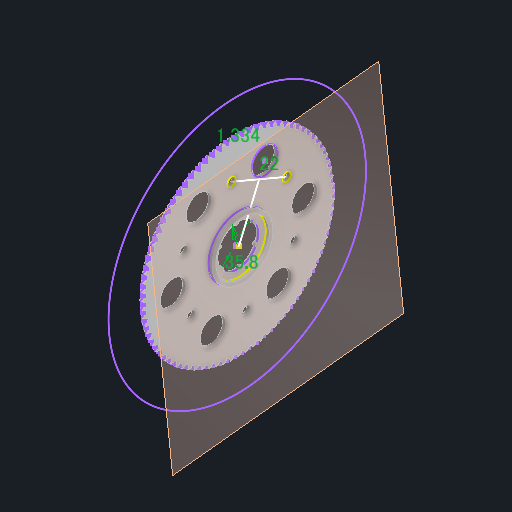
# Autodesk Inventor part: 25A80_()
Saved by Autodesk Inventor 2025.2 (Build 292293000, 293)
## iProperties
Category: PARTsolutions
Company: KANA
Created: 2025-03-15
Part Number: 25A80_()
Material: Generic
Catalog Web Link: www.cadenas.de
Description: 25A-Un-finished
Vendor: KANA
Document SubType Name: Modeling
Designer: psAdmin
Manufacturer: KANA
Mass: 58.7278 g
Surface Area: 427.105 cm^2
Volume: 58.7278 cm^3
Density: 1 g/cm^3
Appearance: PSOLRGB-175-175-175
PSOL_IDENT_0: {$CADENAS_DATA/23d-libs/kana/sprockets/chain_no_25/un_finished_sprocket_steel/a_type/25a.prj},156 {V
PSOL_IDENT_1: TYP=3D},{NB=25A80_()},{LINA=25A80},{NN=25A},{DATE=07.03.2025 00:51:20},{GEOMDATE=20.11.2024 07:31:23
PSOL_IDENT_2: },{VERSION=},{LINEID=550},{WBVAR=SURFT},{WBNUMERIC=}  {NB=25A80_()},{LINA=25A80},{KT=DUMMY},{ORDERNO=
PSOL_IDENT_3: 25A80},{TYPE=25A},{NOT=80},{NOTX=80.000},{DP=161.74},{DC=158.44},{DC2=158.44},{DO=165},{T=2.9},{DR=3
PSOL_IDENT_4: .300},{MAT=None},{MATC=},{SD=11},{SURFT=},{SURFTNB=},{DCX2=0},{CAUTION=The tooth profile in the CAD
PSOL_IDENT_5: models differ from the actual shape.}
NB: 25A80_()
NN: 25A
NT: Un-finished
NBSYN: 25A$NOT._($SURFT.)
LINA: 25A80
CATALOG: KANA
TYPE: 25A
NOT: 80
DP: 161.74
DC: 158.44
DC2: 158.44
DO: 165
T: 2.9
SD: 11
SURFT: No symbol : No
CAUTION: The tooth profile in the CAD models differ from the actual shape.
SUPPLIER: KANA
ARTICLENO: 25A80_()
BOMINFO: 25A80
CREATOR: CADENAS GmbH
Title: 25A80
Author: Cadenas PARTsolutions
Comments: Un-finished
Autodesk Inventor part; units mm, degrees
(part 1 of 2)
ref_plane "YZ Plane" through (0, 0, 0) normal (1, 0, 0) x (0, 1, 0)
ref_plane "XZ Plane" through (0, 0, 0) normal (0, 1, 0) x (-1, 0, 0)
ref_plane "XY Plane" through (0, 0, 0) normal (0, 0, 1) x (1, 0, 0)
sketch "Sketch_1" plane through (0, 0, 0) normal (0, 0, 1) x (1, 0, 0)
  line L0 (2.9, 0) -> (0, 0)
  line L1 (0, 5.5) -> (2.9, 5.5)
  line L2 (2.9, 5.5) -> (2.9, 81.2642)
  arc A0 (2.9, 81.2642) -> (2.175, 82.5) centre (-0.241, 80.2521) ccw
  line L3 (2.175, 82.5) -> (0.725, 82.5)
  arc A1 (0.725, 82.5) -> (0, 81.2642) centre (3.141, 80.2521) ccw
  line L4 (0, 81.2642) -> (0, 5.5)
  constraints: 10 end point, 4 point on circle, 2 centre point
revolve "Revolution1" add sketch "Sketch_1" angle 360 about axis through (2.9, 0, 0) along (1, 0, 0)
sketch "Sketch_2" plane through (1.45, 0, 0) normal (1, 0, 0) x (0, 0, -1)
  circle A0 centre (0, 0) radius 110
  arc A1 (-82.4999, 0.15) -> (-82.4999, -0.15) centre (0, 0) ccw
  line L0 (-82.4999, -0.15) -> (-79.9248, -1.781)
  arc A2 (-79.8181, -4.4953) -> (-79.9248, -1.781) centre (-80.8077, -3.1749) ccw
  line L1 (-79.8181, -4.4953) -> (-82.2573, -6.3233)
  arc A3 (-82.2573, -6.3233) -> (-82.2338, -6.6224) centre (0, 0) ccw
  line L2 (-82.2338, -6.6224) -> (-79.5387, -8.0464)
  arc A4 (-79.2194, -10.7439) -> (-79.5387, -8.0464) centre (-80.3094, -9.5053) ccw
  line L3 (-79.2194, -10.7439) -> (-81.5076, -12.7577)
  arc A5 (-81.5076, -12.7577) -> (-81.4607, -13.054) centre (0, 0) ccw
  line L4 (-81.4607, -13.054) -> (-78.6621, -14.2621)
  arc A6 (-78.1322, -16.9263) -> (-78.6621, -14.2621) centre (-79.3161, -15.777) ccw
  line L5 (-78.1322, -16.9263) -> (-80.2554, -19.1134)
  arc A7 (-80.2554, -19.1134) -> (-80.1854, -19.4051) centre (0, 0) ccw
  line L6 (-80.1854, -19.4051) -> (-77.3007, -20.3899)
  arc A8 (-76.5633, -23.0043) -> (-77.3007, -20.3899) centre (-77.8338, -21.9514) ccw
  line L7 (-76.5633, -23.0043) -> (-78.5084, -25.3512)
  arc A9 (-78.5084, -25.3512) -> (-78.4157, -25.6365) centre (0, 0) ccw
  line L8 (-78.4157, -25.6365) -> (-75.4626, -26.392)
  arc A10 (-74.5224, -28.9404) -> (-75.4626, -26.392) centre (-75.8715, -27.9905) ccw
  line L9 (-74.5224, -28.9404) -> (-76.2773, -31.4328)
  arc A11 (-76.2773, -31.4328) -> (-76.1625, -31.7099) centre (0, 0) ccw
  line L10 (-76.1625, -31.7099) -> (-73.1593, -32.2313)
  arc A12 (-72.0221, -34.6982) -> (-73.1593, -32.2313) centre (-73.4415, -33.857) ccw
  line L11 (-72.0221, -34.6982) -> (-73.576, -37.3205)
  arc A13 (-73.576, -37.3205) -> (-73.4398, -37.5878) centre (0, 0) ccw
  line L12 (-73.4398, -37.5878) -> (-70.4049, -37.872)
  arc A14 (-69.0776, -40.242) -> (-70.4049, -37.872) centre (-70.5588, -39.5148) ccw
  line L13 (-69.0776, -40.242) -> (-70.4211, -42.9782)
  arc A15 (-70.4211, -42.9782) -> (-70.2643, -43.234) centre (0, 0) ccw
  line L14 (-70.2643, -43.234) -> (-67.2165, -43.2791)
  arc A16 (-65.7074, -45.5377) -> (-67.2165, -43.2791) centre (-67.2409, -44.929) ccw
  line L15 (-65.7074, -45.5377) -> (-66.832, -48.3709)
  arc A17 (-66.832, -48.3709) -> (-66.6556, -48.6136) centre (0, 0) ccw
  line L16 (-66.6556, -48.6136) -> (-63.6136, -48.4195)
  arc A18 (-61.932, -50.5527) -> (-63.6136, -48.4195) centre (-63.5086, -50.0661) ccw
  line L17 (-61.932, -50.5527) -> (-62.8308, -53.4653)
  arc A19 (-62.8308, -53.4653) -> (-62.636, -53.6934) centre (0, 0) ccw
  line L18 (-62.636, -53.6934) -> (-59.6186, -53.2613)
  arc A20 (-57.7747, -55.256) -> (-59.6186, -53.2613) centre (-59.3847, -54.8946) ccw
  line L19 (-57.7747, -55.256) -> (-58.4423, -58.2302)
  arc A21 (-58.4423, -58.2302) -> (-58.2301, -58.4423) centre (0, 0) ccw
  line L20 (-58.2301, -58.4423) -> (-55.256, -57.7747)
  arc A22 (-53.2613, -59.6186) -> (-55.256, -57.7747) centre (-54.8946, -59.3847) ccw
  line L21 (-53.2613, -59.6186) -> (-53.6934, -62.636)
  arc A23 (-53.6934, -62.636) -> (-53.4653, -62.8308) centre (0, 0) ccw
  line L22 (-53.4653, -62.8308) -> (-50.5527, -61.932)
  arc A24 (-48.4195, -63.6136) -> (-50.5527, -61.932) centre (-50.0661, -63.5086) ccw
  line L23 (-48.4195, -63.6136) -> (-48.6136, -66.6556)
  arc A25 (-48.6136, -66.6556) -> (-48.3709, -66.832) centre (0, 0) ccw
  line L24 (-48.3709, -66.832) -> (-45.5377, -65.7074)
  arc A26 (-43.2791, -67.2165) -> (-45.5377, -65.7074) centre (-44.929, -67.241) ccw
  line L25 (-43.2791, -67.2165) -> (-43.234, -70.2643)
  arc A27 (-43.234, -70.2643) -> (-42.9782, -70.4211) centre (0, 0) ccw
  line L26 (-42.9782, -70.4211) -> (-40.242, -69.0777)
  arc A28 (-37.872, -70.4049) -> (-40.242, -69.0777) centre (-39.5148, -70.5588) ccw
  line L27 (-37.872, -70.4049) -> (-37.5878, -73.4398)
  arc A29 (-37.5878, -73.4398) -> (-37.3205, -73.576) centre (0, 0) ccw
  line L28 (-37.3205, -73.576) -> (-34.6982, -72.0221)
  arc A30 (-32.2313, -73.1593) -> (-34.6982, -72.0221) centre (-33.857, -73.4415) ccw
  line L29 (-32.2313, -73.1593) -> (-31.7099, -76.1625)
  arc A31 (-31.7099, -76.1625) -> (-31.4327, -76.2773) centre (0, 0) ccw
  line L30 (-31.4327, -76.2773) -> (-28.9404, -74.5224)
  arc A32 (-26.392, -75.4626) -> (-28.9404, -74.5224) centre (-27.9905, -75.8715) ccw
  line L31 (-26.392, -75.4626) -> (-25.6365, -78.4157)
  arc A33 (-25.6365, -78.4157) -> (-25.3512, -78.5084) centre (0, 0) ccw
  line L32 (-25.3512, -78.5084) -> (-23.0043, -76.5633)
  arc A34 (-20.3899, -77.3007) -> (-23.0043, -76.5633) centre (-21.9514, -77.8338) ccw
  line L33 (-20.3899, -77.3007) -> (-19.4051, -80.1854)
  arc A35 (-19.4051, -80.1854) -> (-19.1134, -80.2554) centre (0, 0) ccw
  line L34 (-19.1134, -80.2554) -> (-16.9263, -78.1322)
  arc A36 (-14.2621, -78.6622) -> (-16.9263, -78.1322) centre (-15.777, -79.3161) ccw
  line L35 (-14.2621, -78.6622) -> (-13.054, -81.4607)
  arc A37 (-13.054, -81.4607) -> (-12.7577, -81.5076) centre (0, 0) ccw
  line L36 (-12.7577, -81.5076) -> (-10.7439, -79.2194)
  arc A38 (-8.0464, -79.5387) -> (-10.7439, -79.2194) centre (-9.5052, -80.3095) ccw
  line L37 (-8.0464, -79.5387) -> (-6.6224, -82.2338)
  arc A39 (-6.6224, -82.2338) -> (-6.3233, -82.2573) centre (0, 0) ccw
  line L38 (-6.3233, -82.2573) -> (-4.4953, -79.8181)
  arc A40 (-1.781, -79.9248) -> (-4.4953, -79.8181) centre (-3.1749, -80.8077) ccw
  line L39 (-1.781, -79.9248) -> (-0.15, -82.4999)
  arc A41 (-0.15, -82.4999) -> (0.15, -82.4999) centre (0, 0) ccw
  line L40 (0.15, -82.4999) -> (1.781, -79.9248)
  arc A42 (4.4953, -79.8181) -> (1.781, -79.9248) centre (3.1749, -80.8077) ccw
  line L41 (4.4953, -79.8181) -> (6.3233, -82.2573)
  arc A43 (6.3233, -82.2573) -> (6.6224, -82.2338) centre (0, 0) ccw
  line L42 (6.6224, -82.2338) -> (8.0464, -79.5387)
  arc A44 (10.7439, -79.2194) -> (8.0464, -79.5387) centre (9.5052, -80.3095) ccw
  line L43 (10.7439, -79.2194) -> (12.7577, -81.5076)
  arc A45 (12.7577, -81.5076) -> (13.054, -81.4607) centre (0, 0) ccw
  line L44 (13.054, -81.4607) -> (14.2621, -78.6622)
  arc A46 (16.9263, -78.1322) -> (14.2621, -78.6622) centre (15.777, -79.3161) ccw
  line L45 (16.9263, -78.1322) -> (19.1134, -80.2554)
  arc A47 (19.1134, -80.2554) -> (19.4051, -80.1854) centre (0, 0) ccw
  line L46 (19.4051, -80.1854) -> (20.3899, -77.3007)
  arc A48 (23.0043, -76.5633) -> (20.3899, -77.3007) centre (21.9514, -77.8338) ccw
  line L47 (23.0043, -76.5633) -> (25.3512, -78.5084)
  arc A49 (25.3512, -78.5084) -> (25.6365, -78.4157) centre (0, 0) ccw
  line L48 (25.6365, -78.4157) -> (26.392, -75.4626)
  arc A50 (28.9404, -74.5224) -> (26.392, -75.4626) centre (27.9905, -75.8715) ccw
  line L49 (28.9404, -74.5224) -> (31.4327, -76.2773)
  arc A51 (31.4327, -76.2773) -> (31.7099, -76.1625) centre (0, 0) ccw
  line L50 (31.7099, -76.1625) -> (32.2313, -73.1593)
  arc A52 (34.6982, -72.0221) -> (32.2313, -73.1593) centre (33.857, -73.4415) ccw
  line L51 (34.6982, -72.0221) -> (37.3205, -73.576)
  arc A53 (37.3205, -73.576) -> (37.5878, -73.4398) centre (0, 0) ccw
  line L52 (37.5878, -73.4398) -> (37.872, -70.4049)
  arc A54 (40.242, -69.0777) -> (37.872, -70.4049) centre (39.5148, -70.5588) ccw
  line L53 (40.242, -69.0777) -> (42.9782, -70.4211)
  arc A55 (42.9782, -70.4211) -> (43.234, -70.2643) centre (0, 0) ccw
  line L54 (43.234, -70.2643) -> (43.2791, -67.2165)
  arc A56 (45.5377, -65.7074) -> (43.2791, -67.2165) centre (44.929, -67.241) ccw
  line L55 (45.5377, -65.7074) -> (48.3709, -66.832)
  arc A57 (48.3709, -66.832) -> (48.6136, -66.6556) centre (0, 0) ccw
  line L56 (48.6136, -66.6556) -> (48.4195, -63.6136)
  arc A58 (50.5527, -61.932) -> (48.4195, -63.6136) centre (50.0661, -63.5086) ccw
  line L57 (50.5527, -61.932) -> (53.4653, -62.8308)
  arc A59 (53.4653, -62.8308) -> (53.6934, -62.636) centre (0, 0) ccw
  line L58 (53.6934, -62.636) -> (53.2613, -59.6186)
  arc A60 (55.256, -57.7747) -> (53.2613, -59.6186) centre (54.8946, -59.3847) ccw
  line L59 (55.256, -57.7747) -> (58.2301, -58.4423)
  arc A61 (58.2301, -58.4423) -> (58.4423, -58.2302) centre (0, 0) ccw
  line L60 (58.4423, -58.2302) -> (57.7747, -55.256)
  arc A62 (59.6186, -53.2613) -> (57.7747, -55.256) centre (59.3847, -54.8946) ccw
  line L61 (59.6186, -53.2613) -> (62.636, -53.6934)
  arc A63 (62.636, -53.6934) -> (62.8308, -53.4653) centre (0, 0) ccw
  line L62 (62.8308, -53.4653) -> (61.932, -50.5527)
  arc A64 (63.6136, -48.4195) -> (61.932, -50.5527) centre (63.5086, -50.0661) ccw
  line L63 (63.6136, -48.4195) -> (66.6556, -48.6136)
  arc A65 (66.6556, -48.6136) -> (66.832, -48.3709) centre (0, 0) ccw
  line L64 (66.832, -48.3709) -> (65.7074, -45.5377)
  arc A66 (67.2165, -43.2791) -> (65.7074, -45.5377) centre (67.2409, -44.929) ccw
  line L65 (67.2165, -43.2791) -> (70.2643, -43.234)
  arc A67 (70.2643, -43.234) -> (70.4211, -42.9782) centre (0, 0) ccw
  line L66 (70.4211, -42.9782) -> (69.0776, -40.242)
  arc A68 (70.4049, -37.872) -> (69.0776, -40.242) centre (70.5588, -39.5148) ccw
  line L67 (70.4049, -37.872) -> (73.4398, -37.5878)
  arc A69 (73.4398, -37.5878) -> (73.576, -37.3205) centre (0, 0) ccw
  line L68 (73.576, -37.3205) -> (72.0221, -34.6982)
  arc A70 (73.1593, -32.2313) -> (72.0221, -34.6982) centre (73.4415, -33.857) ccw
  line L69 (73.1593, -32.2313) -> (76.1625, -31.7099)
  arc A71 (76.1625, -31.7099) -> (76.2773, -31.4328) centre (0, 0) ccw
  line L70 (76.2773, -31.4328) -> (74.5224, -28.9404)
  arc A72 (75.4626, -26.392) -> (74.5224, -28.9404) centre (75.8715, -27.9905) ccw
  line L71 (75.4626, -26.392) -> (78.4157, -25.6365)
  arc A73 (78.4157, -25.6365) -> (78.5084, -25.3512) centre (0, 0) ccw
  line L72 (78.5084, -25.3512) -> (76.5633, -23.0043)
  arc A74 (77.3007, -20.3899) -> (76.5633, -23.0043) centre (77.8338, -21.9514) ccw
  line L73 (77.3007, -20.3899) -> (80.1854, -19.4051)
  arc A75 (80.1854, -19.4051) -> (80.2554, -19.1134) centre (0, 0) ccw
  line L74 (80.2554, -19.1134) -> (78.1322, -16.9263)
  arc A76 (78.6621, -14.2621) -> (78.1322, -16.9263) centre (79.3161, -15.777) ccw
  line L75 (78.6621, -14.2621) -> (81.4607, -13.054)
  arc A77 (81.4607, -13.054) -> (81.5076, -12.7577) centre (0, 0) ccw
  line L76 (81.5076, -12.7577) -> (79.2194, -10.7439)
  arc A78 (79.5387, -8.0464) -> (79.2194, -10.7439) centre (80.3094, -9.5053) ccw
  line L77 (79.5387, -8.0464) -> (82.2338, -6.6224)
  arc A79 (82.2338, -6.6224) -> (82.2573, -6.3233) centre (0, 0) ccw
  line L78 (82.2573, -6.3233) -> (79.8181, -4.4953)
  arc A80 (79.9248, -1.781) -> (79.8181, -4.4953) centre (80.8077, -3.1749) ccw
  line L79 (79.9248, -1.781) -> (82.4999, -0.15)
  arc A81 (82.4999, -0.15) -> (82.4999, 0.15) centre (0, 0) ccw
  line L80 (82.4999, 0.15) -> (79.9248, 1.781)
  arc A82 (79.0225, 3.671) -> (79.9248, 1.781) centre (80.6244, 3.2753) ccw
  line L81 (79.0225, 3.671) -> (81.4805, 5.4737)
  arc A83 (81.4805, 5.4737) -> (81.46, 5.773) centre (-0.8378, 0.0009) ccw
  line L82 (81.46, 5.773) -> (78.7798, 7.2248)
  arc A84 (78.4884, 9.9255) -> (78.7798, 7.2248) centre (79.5656, 8.6756) ccw
  line L83 (78.4884, 9.9255) -> (80.7973, 11.9155)
  arc A85 (80.7973, 11.9155) -> (80.7535, 12.2122) centre (-0.8378, 0.0009) ccw
  line L84 (80.7535, 12.2122) -> (77.9676, 13.4492)
  arc A86 (77.4652, 16.1187) -> (77.9676, 13.4492) centre (78.6371, 14.9572) ccw
  line L85 (77.4652, 16.1187) -> (79.6109, 18.2838)
  arc A87 (79.6109, 18.2838) -> (79.5439, 18.5762) centre (-0.8378, 0.0009) ccw
  line L86 (79.5439, 18.5762) -> (76.6695, 19.5908)
  arc A88 (75.9592, 22.2126) -> (76.6695, 19.5908) centre (77.2187, 21.1467) ccw
  line L87 (75.9592, 22.2126) -> (77.9284, 24.5393)
  arc A89 (77.9284, 24.5393) -> (77.8387, 24.8256) centre (-0.8378, 0.0009) ccw
  line L88 (77.8387, 24.8256) -> (74.8936, 25.6115)
  arc A90 (73.9798, 28.1696) -> (74.8936, 25.6115) centre (75.319, 27.2057) ccw
  line L89 (73.9798, 28.1696) -> (75.7604, 30.6436)
  arc A91 (75.7604, 30.6436) -> (75.6484, 30.9219) centre (-0.8378, 0.0009) ccw
  line L90 (75.6484, 30.9219) -> (72.6507, 31.4744)
  arc A92 (71.539, 33.9529) -> (72.6507, 31.4744) centre (72.9498, 33.0971) ccw
  line L91 (71.539, 33.9529) -> (73.12, 36.559)
  arc A93 (73.12, 36.559) -> (72.9866, 36.8277) centre (-0.8378, 0.0009) ccw
  line L92 (72.9866, 36.8277) -> (69.9548, 37.1432)
  arc A94 (68.6521, 39.5268) -> (69.9548, 37.1432) centre (70.1256, 38.7843) ccw
  line L93 (68.6521, 39.5268) -> (70.0237, 42.2489)
  arc A95 (70.0237, 42.2489) -> (69.8696, 42.5063) centre (-0.8378, 0.0009) ccw
  line L94 (69.8696, 42.5063) -> (66.8224, 42.583)
  arc A96 (65.3367, 44.8571) -> (66.8224, 42.583) centre (66.8639, 44.2325) ccw
  line L95 (65.3367, 44.8571) -> (66.4905, 47.6784)
  arc A97 (66.4905, 47.6784) -> (66.3167, 47.9229) centre (-0.8378, 0.0009) ccw
  line L96 (66.3167, 47.9229) -> (63.2729, 47.7603)
  arc A98 (61.6133, 49.9108) -> (63.2729, 47.7603) centre (63.1849, 49.408) ccw
  line L97 (61.6133, 49.9108) -> (62.5425, 52.8149)
  arc A99 (62.5425, 52.8149) -> (62.3498, 53.0441) centre (-0.5024, 0) ccw
  line L98 (62.3498, 53.0441) -> (59.3281, 52.6432)
  arc A100 (57.5049, 54.6568) -> (59.3281, 52.6432) centre (59.1111, 54.2788) ccw
  line L99 (57.5049, 54.6568) -> (58.2032, 57.6239)
  arc A101 (58.2032, 57.6239) -> (57.9933, 57.8382) centre (-0.8378, 0.0009) ccw
  line L100 (57.9933, 57.8382) -> (55.0124, 57.2014)
  arc A102 (53.0368, 59.0658) -> (55.0124, 57.2014) centre (54.6677, 58.815) ccw
  line L101 (53.0368, 59.0658) -> (53.5002, 62.0786)
  arc A103 (53.5002, 62.0786) -> (53.2741, 62.2758) centre (-0.8378, 0.0009) ccw
  line L102 (53.2741, 62.2758) -> (50.3523, 61.4071)
  arc A104 (48.2366, 63.1107) -> (50.3523, 61.4071) centre (49.8821, 62.9886) ccw
  line L103 (48.2366, 63.1107) -> (48.4621, 66.1505)
  arc A105 (48.4621, 66.1505) -> (48.2212, 66.3294) centre (-0.8378, 0.0009) ccw
  line L104 (48.2212, 66.3294) -> (45.3766, 65.2341)
  arc A106 (43.1338, 66.7665) -> (45.3766, 65.2341) centre (44.7837, 66.7739) ccw
  line L105 (43.1338, 66.7665) -> (43.1201, 69.8146)
  arc A107 (43.1201, 69.8146) -> (42.8659, 69.974) centre (-0.8378, 0.0009) ccw
  line L106 (42.8659, 69.974) -> (40.116, 68.6589)
  arc A108 (37.7598, 70.0106) -> (40.116, 68.6589) centre (39.4042, 70.1475) ccw
  line L107 (37.7598, 70.0106) -> (37.507, 73.0483)
  arc A109 (37.507, 73.0483) -> (37.2412, 73.1873) centre (-0.8378, 0.0009) ccw
  line L108 (37.2412, 73.1873) -> (34.6029, 71.6605)
  arc A110 (32.148, 72.8232) -> (34.6029, 71.6605) centre (33.7765, 73.0886) ccw
  line L109 (32.148, 72.8232) -> (31.6576, 75.8316)
  arc A111 (31.6576, 75.8316) -> (31.3816, 75.9493) centre (-0.8378, 0.0009) ccw
  line L110 (31.3816, 75.9493) -> (28.8713, 74.2202)
  arc A112 (26.3327, 75.1867) -> (28.8713, 74.2202) centre (27.9354, 75.5791) ccw
  line L111 (26.3327, 75.1867) -> (25.6078, 78.1474)
  arc A113 (25.6078, 78.1474) -> (25.3235, 78.2431) centre (-0.8378, 0.0009) ccw
  line L112 (25.3235, 78.2431) -> (22.9566, 76.3224)
  arc A114 (20.3499, 77.0867) -> (22.9566, 76.3224) centre (21.9169, 77.6036) ccw
  line L113 (20.3499, 77.0867) -> (19.395, 79.9814)
  arc A115 (19.395, 79.9814) -> (19.104, 80.0545) centre (-0.8378, 0.0009) ccw
  line L114 (19.104, 80.0545) -> (16.8951, 77.954)
  arc A116 (14.2365, 78.5114) -> (16.8951, 77.954) centre (15.7581, 79.1497) ccw
  line L115 (14.2365, 78.5114) -> (13.0574, 81.3223)
  arc A117 (13.0574, 81.3223) -> (12.7616, 81.3723) centre (-0.8378, 0.0009) ccw
  line L116 (12.7616, 81.3723) -> (10.7243, 79.105)
  arc A118 (8.0302, 79.4521) -> (10.7243, 79.105) centre (9.497, 80.2078) ccw
  line L117 (8.0302, 79.4521) -> (6.6342, 82.1618)
  arc A119 (6.6342, 82.1618) -> (6.3354, 82.1885) centre (-0.8378, 0.0009) ccw
  line L118 (6.3354, 82.1885) -> (4.4822, 79.7683)
  arc A120 (1.7692, 79.903) -> (4.4822, 79.7683) centre (3.1722, 80.7714) ccw
  line L119 (1.7692, 79.903) -> (0.1649, 82.4948)
  arc A121 (0.1649, 82.4948) -> (-0.15, 82.4999) centre (-1.3174, 0.0081) ccw
  line L120 (-0.15, 82.4999) -> (-1.781, 79.9248)
  arc A122 (-4.4953, 79.8181) -> (-1.781, 79.9248) centre (-3.1749, 80.8077) ccw
  line L121 (-4.4953, 79.8181) -> (-6.3233, 82.2573)
  arc A123 (-6.3233, 82.2573) -> (-6.6224, 82.2338) centre (0, 0) ccw
  line L122 (-6.6224, 82.2338) -> (-8.0464, 79.5386)
  arc A124 (-10.7439, 79.2194) -> (-8.0464, 79.5386) centre (-9.5052, 80.3094) ccw
  line L123 (-10.7439, 79.2194) -> (-12.7577, 81.5076)
  arc A125 (-12.7577, 81.5076) -> (-13.054, 81.4607) centre (0, 0) ccw
  line L124 (-13.054, 81.4607) -> (-14.2621, 78.6621)
  arc A126 (-16.9263, 78.1322) -> (-14.2621, 78.6621) centre (-15.777, 79.3161) ccw
  line L125 (-16.9263, 78.1322) -> (-19.1134, 80.2554)
  arc A127 (-19.1134, 80.2554) -> (-19.4051, 80.1854) centre (0, 0) ccw
  line L126 (-19.4051, 80.1854) -> (-20.3899, 77.3007)
  arc A128 (-23.0043, 76.5633) -> (-20.3899, 77.3007) centre (-21.9514, 77.8338) ccw
  line L127 (-23.0043, 76.5633) -> (-25.3512, 78.5084)
  arc A129 (-25.3512, 78.5084) -> (-25.6365, 78.4157) centre (0, 0) ccw
  line L128 (-25.6365, 78.4157) -> (-26.392, 75.4626)
  arc A130 (-28.9404, 74.5224) -> (-26.392, 75.4626) centre (-27.9905, 75.8715) ccw
  line L129 (-28.9404, 74.5224) -> (-31.4327, 76.2773)
  arc A131 (-31.4327, 76.2773) -> (-31.7099, 76.1625) centre (0, 0) ccw
  line L130 (-31.7099, 76.1625) -> (-32.2313, 73.1593)
  arc A132 (-34.6982, 72.0221) -> (-32.2313, 73.1593) centre (-33.857, 73.4415) ccw
  line L131 (-34.6982, 72.0221) -> (-37.3205, 73.576)
  arc A133 (-37.3205, 73.576) -> (-37.5878, 73.4398) centre (0, 0) ccw
  line L132 (-37.5878, 73.4398) -> (-37.872, 70.4049)
  arc A134 (-40.242, 69.0776) -> (-37.872, 70.4049) centre (-39.5148, 70.5588) ccw
  line L133 (-40.242, 69.0776) -> (-42.9782, 70.4211)
  arc A135 (-42.9782, 70.4211) -> (-43.234, 70.2643) centre (0, 0) ccw
  line L134 (-43.234, 70.2643) -> (-43.2791, 67.2165)
  arc A136 (-45.5377, 65.7074) -> (-43.2791, 67.2165) centre (-44.929, 67.2409) ccw
  line L135 (-45.5377, 65.7074) -> (-48.3709, 66.832)
  arc A137 (-48.3709, 66.832) -> (-48.6136, 66.6556) centre (0, 0) ccw
  line L136 (-48.6136, 66.6556) -> (-48.4195, 63.6136)
  arc A138 (-50.5527, 61.9319) -> (-48.4195, 63.6136) centre (-50.0661, 63.5086) ccw
  line L137 (-50.5527, 61.9319) -> (-53.4653, 62.8308)
  arc A139 (-53.4653, 62.8308) -> (-53.6934, 62.636) centre (0, 0) ccw
  line L138 (-53.6934, 62.636) -> (-53.2613, 59.6186)
  arc A140 (-55.256, 57.7747) -> (-53.2613, 59.6186) centre (-54.8946, 59.3847) ccw
  line L139 (-55.256, 57.7747) -> (-58.2301, 58.4423)
  arc A141 (-58.2301, 58.4423) -> (-58.4423, 58.2301) centre (0, 0) ccw
  line L140 (-58.4423, 58.2301) -> (-57.7747, 55.256)
  arc A142 (-59.6186, 53.2613) -> (-57.7747, 55.256) centre (-59.3847, 54.8946) ccw
  line L141 (-59.6186, 53.2613) -> (-62.636, 53.6934)
  arc A143 (-62.636, 53.6934) -> (-62.8308, 53.4653) centre (0, 0) ccw
  line L142 (-62.8308, 53.4653) -> (-61.932, 50.5527)
  arc A144 (-63.6136, 48.4195) -> (-61.932, 50.5527) centre (-63.5086, 50.0661) ccw
  line L143 (-63.6136, 48.4195) -> (-66.6556, 48.6136)
  arc A145 (-66.6556, 48.6136) -> (-66.832, 48.3708) centre (0, 0) ccw
  line L144 (-66.832, 48.3708) -> (-65.7074, 45.5377)
  arc A146 (-67.2165, 43.2791) -> (-65.7074, 45.5377) centre (-67.2409, 44.929) ccw
  line L145 (-67.2165, 43.2791) -> (-70.2643, 43.234)
  arc A147 (-70.2643, 43.234) -> (-70.4211, 42.9782) centre (0, 0) ccw
  line L146 (-70.4211, 42.9782) -> (-69.0776, 40.242)
  arc A148 (-70.4049, 37.872) -> (-69.0776, 40.242) centre (-70.5588, 39.5148) ccw
  line L147 (-70.4049, 37.872) -> (-73.4398, 37.5878)
  arc A149 (-73.4398, 37.5878) -> (-73.576, 37.3205) centre (0, 0) ccw
  line L148 (-73.576, 37.3205) -> (-72.0221, 34.6982)
  arc A150 (-73.1593, 32.2313) -> (-72.0221, 34.6982) centre (-73.4415, 33.857) ccw
  line L149 (-73.1593, 32.2313) -> (-76.1625, 31.7099)
  arc A151 (-76.1625, 31.7099) -> (-76.2773, 31.4327) centre (0, 0) ccw
  line L150 (-76.2773, 31.4327) -> (-74.5224, 28.9404)
  arc A152 (-75.4626, 26.392) -> (-74.5224, 28.9404) centre (-75.8715, 27.9905) ccw
  line L151 (-75.4626, 26.392) -> (-78.4157, 25.6365)
  arc A153 (-78.4157, 25.6365) -> (-78.5084, 25.3512) centre (0, 0) ccw
  line L152 (-78.5084, 25.3512) -> (-76.5633, 23.0043)
  arc A154 (-77.3007, 20.3899) -> (-76.5633, 23.0043) centre (-77.8338, 21.9514) ccw
  line L153 (-77.3007, 20.3899) -> (-80.1854, 19.4051)
  arc A155 (-80.1854, 19.4051) -> (-80.2554, 19.1134) centre (0, 0) ccw
  line L154 (-80.2554, 19.1134) -> (-78.1322, 16.9263)
  arc A156 (-78.6621, 14.2621) -> (-78.1322, 16.9263) centre (-79.3161, 15.777) ccw
  line L155 (-78.6621, 14.2621) -> (-81.4607, 13.054)
  arc A157 (-81.4607, 13.054) -> (-81.5076, 12.7577) centre (0, 0) ccw
  line L156 (-81.5076, 12.7577) -> (-79.2194, 10.7439)
  arc A158 (-79.5387, 8.0464) -> (-79.2194, 10.7439) centre (-80.3094, 9.5052) ccw
  line L157 (-79.5387, 8.0464) -> (-82.2338, 6.6224)
  arc A159 (-82.2338, 6.6224) -> (-82.2573, 6.3233) centre (0, 0) ccw
  line L158 (-82.2573, 6.3233) -> (-79.8181, 4.4953)
  arc A160 (-79.9248, 1.781) -> (-79.8181, 4.4953) centre (-80.8077, 3.1749) ccw
  line L159 (-79.9248, 1.781) -> (-82.4999, 0.15)
  arc A161 (0.667, 81.6835) -> (-0.667, 81.6835) centre (0, 0) ccw
  circle A162 centre (0, 0) radius 17.9
  line L160 (-0.3663, 82.1584) -> (0.3731, 82.1584)
  dimension "d5" = 1.3341
  dimension "d19" = 35.8
  constraints: 322 end point, 322 point on circle, 163 centre point, 4 point on line, 2 coincident, 1 horizontal
  measures "d5" distance of A161.start A161.end
  measures "d19" diameter of A162
extrude "Extrusion1" cut sketch "Sketch_2" along normal mid plane 3.3 contours A0
ref_plane "Body_XY" through (0, 0, 0) normal (1, 0, 0) x (0, 0, -1)
ref_plane "Body_YZ" through (0, 0, 0) normal (0, 0, -1) x (0, 1, 0)
ref_plane "Body_ZX" through (0, 0, 0) normal (0, 1, 0) x (1, 0, 0)
sketch "スケッチ3" plane through (2.9, 8.6756, -79.5656) normal (1, 0, 0) x (0, 0.1072674, -0.9942302)
  circle A0 centre (-80.0371, -0.0908) radius 5.5 projected
  line L0 (-1.0768, -4.9175) -> (1.1501, -3.6267) projected
  arc A1 (1.1501, -3.6267) -> (1.1812, -2.8194) centre (-80.0371, -0.0908) ccw projected
  line L1 (1.1812, -2.8194) -> (-0.9369, -1.3582) projected
  arc A2 (-0.9369, 1.3582) -> (-0.9369, -1.3582) centre (0, 0) ccw projected
  line L2 (-0.9369, 1.3582) -> (1.1751, 2.8151) projected
  arc A3 (1.1751, 2.8151) -> (1.1417, 3.6315) centre (-80.0371, -0.0908) ccw projected
  line L3 (1.1417, 3.6315) -> (-1.0768, 4.9175) projected
  arc A4 (-1.2899, 7.6255) -> (-1.0768, 4.9175) centre (-0.2493, 6.345) ccw projected
  line L4 (-1.2899, 7.6255) -> (0.6902, 9.2346) projected
  arc A5 (0.6902, 9.2346) -> (0.5904, 10.0614) centre (-80.0371, -0.0908) ccw projected
  line L5 (0.5904, 10.0614) -> (-1.7086, 11.1628) projected
  arc A6 (-2.1335, 13.8457) -> (-1.7086, 11.1628) centre (-0.9956, 12.6509) ccw projected
  line L6 (-2.1335, 13.8457) -> (-0.3005, 15.5913) projected
  arc A7 (-0.3005, 15.5913) -> (-0.4698, 16.4293) centre (-80.0371, -0.0908) ccw projected
  line L7 (-0.4698, 16.4293) -> (-2.8284, 17.3393) projected
  arc A8 (-3.4625, 19.9807) -> (-2.8284, 17.3393) centre (-2.2344, 18.8787) ccw projected
  line L8 (-3.4625, 19.9807) -> (-1.7896, 21.8452) projected
  arc A9 (-1.7896, 21.8452) -> (-2.0327, 22.6945) centre (-80.0371, -0.0908) ccw projected
  line L9 (-2.0327, 22.6945) -> (-4.4294, 23.409) projected
  arc A10 (-5.2688, 25.9924) -> (-4.4294, 23.409) centre (-3.9581, 24.9902) ccw projected
  line L10 (-5.2688, 25.9924) -> (-3.7667, 27.9571) projected
  arc A11 (-3.7667, 27.9571) -> (-4.0884, 28.8169) centre (-80.0371, -0.0908) ccw projected
  line L11 (-4.0884, 28.8169) -> (-6.5017, 29.3343) projected
  arc A12 (-7.5412, 31.8439) -> (-6.5017, 29.3343) centre (-6.1559, 30.9476) ccw projected
  line L12 (-7.5412, 31.8439) -> (-6.2182, 33.889) projected
  arc A13 (-6.2182, 33.889) -> (-6.6241, 34.7574) centre (-80.0371, -0.0908) ccw projected
  line L13 (-6.6241, 34.7574) -> (-9.0325, 35.0787) projected
  arc A14 (-10.2657, 37.499) -> (-9.0325, 35.0787) centre (-8.8143, 36.7142) ccw projected
  line L14 (-10.2657, 37.499) -> (-9.1275, 39.6041) projected
  arc A15 (-9.1275, 39.6041) -> (-9.6237, 40.4779) centre (-80.0371, -0.0908) ccw projected
  line L15 (-9.6237, 40.4779) -> (-12.0062, 40.6069) projected
  arc A16 (-13.4255, 42.923) -> (-12.0062, 40.6069) centre (-11.917, 42.2545) ccw projected
  line L16 (-13.4255, 42.923) -> (-12.4752, 45.0673) projected
  arc A17 (-12.4752, 45.0673) -> (-13.068, 45.9418) centre (-80.0371, -0.0908) ccw projected
  line L17 (-13.068, 45.9418) -> (-15.4045, 45.8847) projected
  arc A18 (-17.0011, 48.0823) -> (-15.4045, 45.8847) centre (-15.4448, 47.5342) ccw projected
  line L18 (-17.0011, 48.0823) -> (-16.2394, 50.2452) projected
  arc A19 (-16.2394, 50.2452) -> (-16.9348, 51.1144) centre (-80.0371, -0.0908) ccw projected
  line L19 (-16.9348, 51.1144) -> (-19.2063, 50.8796) projected
  arc A20 (-20.9705, 52.9451) -> (-19.2063, 50.8796) centre (-19.376, 52.5209) ccw projected
  line L20 (-20.9705, 52.9451) -> (-20.3954, 55.1064) projected
  arc A21 (-20.3954, 55.1064) -> (-21.1994, 55.9626) centre (-80.0371, -0.0908) ccw projected
  line L21 (-21.1994, 55.9626) -> (-23.3884, 55.5608) projected
  arc A22 (-25.3092, 57.4816) -> (-23.3884, 55.5608) centre (-23.6863, 57.1837) ccw projected
  line L22 (-25.3092, 57.4816) -> (-24.9164, 59.6216) projected
  arc A23 (-24.9164, 59.6216) -> (-25.8341, 60.4559) centre (-80.0371, -0.0908) ccw projected
  line L23 (-25.8341, 60.4559) -> (-27.9249, 59.8995) projected
  arc A24 (-29.9904, 61.6637) -> (-27.9249, 59.8995) centre (-28.3491, 61.494) ccw projected
  line L24 (-29.9904, 61.6637) -> (-29.7733, 63.7639) projected
  arc A25 (-29.7733, 63.7639) -> (-30.809, 64.5657) centre (-80.0371, -0.0908) ccw projected
  line L25 (-30.809, 64.5657) -> (-32.7877, 63.8689) projected
  arc A26 (-34.9853, 65.4655) -> (-32.7877, 63.8689) centre (-33.3358, 65.4252) ccw projected
  line L26 (-34.9853, 65.4655) -> (-34.9354, 67.5088) projected
  arc A27 (-34.9354, 67.5088) -> (-36.0922, 68.2665) centre (-80.0371, -0.0908) ccw projected
  line L27 (-36.0922, 68.2665) -> (-37.947, 67.4445) projected
  arc A28 (-40.2631, 68.8638) -> (-37.947, 67.4445) centre (-38.6155, 68.953) ccw projected
  line L28 (-40.2631, 68.8638) -> (-40.3698, 70.8343) projected
  arc A29 (-40.3698, 70.8343) -> (-41.6496, 71.5351) centre (-80.0371, -0.0908) ccw projected
  line L29 (-41.6496, 71.5351) -> (-43.371, 70.6043) projected
  arc A30 (-45.7913, 71.8375) -> (-43.371, 70.6043) centre (-44.1558, 72.0557) ccw projected
  line L30 (-45.7913, 71.8375) -> (-46.0427, 73.7214) projected
  arc A31 (-46.0427, 73.7214) -> (-47.4454, 74.3514) centre (-80.0371, -0.0908) ccw projected
  line L31 (-47.4454, 74.3514) -> (-49.0261, 73.3288) projected
  arc A32 (-51.5357, 74.3683) -> (-49.0261, 73.3288) centre (-49.9224, 74.7141) ccw projected
  line L32 (-51.5357, 74.3683) -> (-51.9185, 76.1536) projected
  arc A33 (-51.9185, 76.1536) -> (-53.4424, 76.6985) centre (-80.0371, -0.0908) ccw projected
  line L33 (-53.4424, 76.6985) -> (-54.8776, 75.6012) projected
  arc A34 (-57.461, 76.4406) -> (-54.8776, 75.6012) centre (-55.8798, 76.9119) ccw projected
  line L34 (-57.461, 76.4406) -> (-57.9609, 78.1173) projected
  arc A35 (-57.9609, 78.1173) -> (-59.6024, 78.5622) centre (-80.0371, -0.0908) ccw projected
  line L35 (-59.6024, 78.5622) -> (-60.8893, 77.4075) projected
  arc A36 (-63.5307, 78.0416) -> (-60.8893, 77.4075) centre (-61.9913, 78.6356) ccw projected
  line L36 (-63.5307, 78.0416) -> (-64.1327, 79.6019) projected
  arc A37 (-64.1327, 79.6019) -> (-65.886, 79.9318) centre (-80.0371, -0.0908) ccw projected
  line L37 (-65.886, 79.9318) -> (-67.0243, 78.7365) projected
  arc A38 (-69.7072, 79.1614) -> (-67.0243, 78.7365) centre (-68.2191, 79.8744) ccw projected
  line L38 (-69.7072, 79.1614) -> (-70.3962, 80.5995) projected
  arc A39 (-70.3962, 80.5995) -> (-72.2514, 80.7996) centre (-80.0371, -0.0908) ccw projected
  line L39 (-72.2514, 80.7996) -> (-73.2346, 79.5639) projected
  arc A40 (-75.9446, 79.749) -> (-73.2346, 79.5639) centre (-74.5257, 80.5912) ccw projected
  line L40 (-75.9446, 79.749) -> (-76.7506, 81.1069) projected
  arc A41 (-76.7506, 81.1069) -> (-78.622, 81.1611) centre (-80.0371, -0.0908) ccw projected
  line L41 (-78.622, 81.1611) -> (-79.5052, 79.8521) projected
  arc A42 (-82.2214, 79.824) -> (-79.5052, 79.8521) centre (-80.873, 80.7749) ccw projected
  line L42 (-82.2214, 79.824) -> (-83.1315, 81.1145) projected
  arc A43 (-83.1315, 81.1145) -> (-85.0013, 81.0217) centre (-80.0371, -0.0908) ccw projected
  line L43 (-85.0013, 81.0217) -> (-85.7791, 79.6474) projected
  arc A44 (-88.4847, 79.4063) -> (-85.7791, 79.6474) centre (-87.215, 80.4601) ccw projected
  line L44 (-88.4847, 79.4063) -> (-89.4932, 80.6214) projected
  arc A45 (-89.4932, 80.6214) -> (-91.35, 80.3821) centre (-80.0371, -0.0908) ccw projected
  line L45 (-91.35, 80.3821) -> (-92.0175, 78.9511) projected
  arc A46 (-94.6959, 78.4984) -> (-92.0175, 78.9511) centre (-93.5129, 79.6486) ccw projected
  line L46 (-94.6959, 78.4984) -> (-95.7967, 79.6307) projected
  arc A47 (-95.7967, 79.6307) -> (-97.629, 79.2465) centre (-80.0371, -0.0908) ccw projected
  line L47 (-97.629, 79.2465) -> (-98.1822, 77.7674) projected
  arc A48 (-100.8168, 77.106) -> (-98.1822, 77.7674) centre (-99.7276, 78.3455) ccw projected
  line L48 (-100.8168, 77.106) -> (-102.0029, 78.1484) projected
  arc A49 (-102.0029, 78.1484) -> (-103.7995, 77.6217) centre (-80.0371, -0.0908) ccw projected
  line L49 (-103.7995, 77.6217) -> (-104.2349, 76.1038) projected
  arc A50 (-106.8095, 75.2377) -> (-104.2349, 76.1038) centre (-105.8209, 76.5588) ccw projected
  line L50 (-106.8095, 75.2377) -> (-108.0738, 76.1838) projected
  arc A51 (-108.0738, 76.1838) -> (-109.8235, 75.5177) centre (-80.0371, -0.0908) ccw projected
  line L51 (-109.8235, 75.5177) -> (-110.1385, 73.9704) projected
  arc A52 (-112.6372, 72.905) -> (-110.1385, 73.9704) centre (-111.7553, 74.2995) ccw projected
  line L52 (-112.6372, 72.905) -> (-113.9718, 73.749) projected
  arc A53 (-113.9718, 73.749) -> (-115.6638, 72.9476) centre (-80.0371, -0.0908) ccw projected
  line L53 (-115.6638, 72.9476) -> (-115.8564, 71.3803) projected
  arc A54 (-118.2639, 70.1222) -> (-115.8564, 71.3803) centre (-117.4941, 71.5816) ccw projected
  line L54 (-118.2639, 70.1222) -> (-119.6606, 70.8589) projected
  arc A55 (-119.6606, 70.8589) -> (-121.2845, 69.9273) centre (-80.0371, -0.0908) ccw projected
  line L55 (-121.2845, 69.9273) -> (-121.3536, 68.3497) projected
  arc A56 (-123.6549, 66.9065) -> (-121.3536, 68.3497) centre (-123.002, 68.4219) ccw projected
  line L56 (-123.6549, 66.9065) -> (-125.1051, 67.5313) projected
  arc A57 (-125.1051, 67.5313) -> (-126.6509, 66.4752) centre (-80.0371, -0.0908) ccw projected
  line L57 (-126.6509, 66.4752) -> (-126.596, 64.897) projected
  arc A58 (-128.777, 63.2778) -> (-126.596, 64.897) centre (-128.245, 64.8397) ccw projected
  line L58 (-128.777, 63.2778) -> (-130.2717, 63.7869) projected
  arc A59 (-130.2717, 63.7869) -> (-131.7299, 62.6127) centre (-80.0371, -0.0908) ccw projected
  line L59 (-131.7299, 62.6127) -> (-131.5514, 61.0437) projected
  arc A60 (-133.5986, 59.2583) -> (-131.5514, 61.0437) centre (-133.1908, 60.8572) ccw projected
  line L60 (-133.5986, 59.2583) -> (-135.1287, 59.6486) projected
  arc A61 (-135.1287, 59.6486) -> (-136.4902, 58.3636) centre (-80.0371, -0.0908) ccw projected
  line L61 (-136.4902, 58.3636) -> (-136.1891, 56.8135) projected
  arc A62 (-138.0899, 54.873) -> (-136.1891, 56.8135) centre (-137.8088, 56.4989) ccw projected
  line L62 (-138.0899, 54.873) -> (-139.6459, 55.142) projected
  arc A63 (-139.6459, 55.142) -> (-140.9025, 53.7542) centre (-80.0371, -0.0908) ccw projected
  line L63 (-140.9025, 53.7542) -> (-140.4807, 52.2325) projected
  arc A64 (-142.2234, 50.1488) -> (-140.4807, 52.2325) centre (-142.0707, 51.7917) ccw projected
  line L64 (-142.2234, 50.1488) -> (-143.7957, 50.2949) projected
  arc A65 (-143.7957, 50.2949) -> (-144.9395, 48.8128) centre (-80.0371, -0.0908) ccw projected
  line L65 (-144.9395, 48.8128) -> (-144.3996, 47.3288) projected
  arc A66 (-145.9734, 45.1149) -> (-144.3996, 47.3288) centre (-145.9501, 46.7647) ccw projected
  line L66 (-145.9734, 45.1149) -> (-147.5524, 45.1371) projected
  arc A67 (-147.5524, 45.1371) -> (-148.5763, 43.5698) centre (-80.0371, -0.0908) ccw projected
  line L67 (-148.5763, 43.5698) -> (-147.9217, 42.1328) projected
  arc A68 (-149.317, 39.8022) -> (-147.9217, 42.1328) centre (-149.4232, 41.4488) ccw projected
  line L68 (-149.317, 39.8022) -> (-150.8928, 39.7005) projected
  arc A69 (-150.8928, 39.7005) -> (-151.7906, 38.0577) centre (-80.0371, -0.0908) ccw projected
  line L69 (-151.7906, 38.0577) -> (-151.0252, 36.6765) projected
  arc A70 (-152.2334, 34.2436) -> (-151.0252, 36.6765) centre (-152.4685, 35.8768) ccw projected
  line L70 (-152.2334, 34.2436) -> (-153.7963, 34.0186) projected
  arc A71 (-153.7963, 34.0186) -> (-154.5625, 32.3104) centre (-80.0371, -0.0908) ccw projected
  line L71 (-154.5625, 32.3104) -> (-153.6911, 30.9935) projected
  arc A72 (-154.7046, 28.4733) -> (-153.6911, 30.9935) centre (-155.0672, 30.083) ccw projected
  line L72 (-154.7046, 28.4733) -> (-156.2452, 28.1264) projected
  arc A73 (-156.2452, 28.1264) -> (-156.8749, 26.3633) centre (-80.0371, -0.0908) ccw projected
  line L73 (-156.8749, 26.3633) -> (-155.9029, 25.1189) projected
  arc A74 (-156.7156, 22.5269) -> (-155.9029, 25.1189) centre (-157.2033, 24.1032) ccw projected
  line L74 (-156.7156, 22.5269) -> (-158.2241, 22.0602) projected
  arc A75 (-158.2241, 22.0602) -> (-158.7136, 20.2532) centre (-80.0371, -0.0908) ccw projected
  line L75 (-158.7136, 20.2532) -> (-157.647, 19.0888) projected
  arc A76 (-158.2538, 16.4411) -> (-157.647, 19.0888) centre (-158.8636, 17.9742) ccw projected
  line L76 (-158.2538, 16.4411) -> (-159.721, 15.8574) projected
  arc A77 (-159.721, 15.8574) -> (-160.0673, 14.0176) centre (-80.0371, -0.0908) ccw projected
  line L77 (-160.0673, 14.0176) -> (-158.9125, 12.9405) projected
  arc A78 (-159.3097, 10.2533) -> (-158.9125, 12.9405) centre (-160.038, 11.7339) ccw projected
  line L78 (-159.3097, 10.2533) -> (-160.7267, 9.5563) projected
  arc A79 (-160.7267, 9.5563) -> (-160.9275, 7.695) centre (-80.0371, -0.0908) ccw projected
  line L79 (-160.9275, 7.695) -> (-159.6918, 6.7118) projected
  arc A80 (-159.8769, 4.0018) -> (-159.6918, 6.7118) centre (-160.7191, 5.4206) ccw projected
  line L80 (-159.8769, 4.0018) -> (-161.2348, 3.1958) projected
  arc A81 (-161.2348, 3.1958) -> (-161.289, 1.3244) centre (-80.0371, -0.0908) ccw projected
  line L81 (-161.289, 1.3244) -> (-159.98, 0.4412) projected
  arc A82 (-159.9519, -2.275) -> (-159.98, 0.4412) centre (-160.9028, -0.9266) ccw projected
  line L82 (-159.9519, -2.275) -> (-161.2424, -3.1851) projected
  arc A83 (-161.2424, -3.1851) -> (-161.1496, -5.0549) centre (-80.0371, -0.0908) ccw projected
  line L83 (-161.1496, -5.0549) -> (-159.7753, -5.8327) projected
  arc A84 (-159.5342, -8.5383) -> (-159.7753, -5.8327) centre (-160.588, -7.2687) ccw projected
  line L84 (-159.5342, -8.5383) -> (-160.7493, -9.5468) projected
  arc A85 (-160.7493, -9.5468) -> (-160.51, -11.4036) centre (-80.0371, -0.0908) ccw projected
  line L85 (-160.51, -11.4036) -> (-159.079, -12.0712) projected
  arc A86 (-158.6263, -14.7495) -> (-159.079, -12.0712) centre (-159.7765, -13.5665) ccw projected
  line L86 (-158.6263, -14.7495) -> (-159.7586, -15.8503) projected
  arc A87 (-159.7586, -15.8503) -> (-159.3744, -17.6826) centre (-80.0371, -0.0908) ccw projected
  line L87 (-159.3744, -17.6826) -> (-157.8953, -18.2358) projected
  arc A88 (-157.234, -20.8704) -> (-157.8953, -18.2358) centre (-158.4734, -19.7812) ccw projected
  line L88 (-157.234, -20.8704) -> (-158.2763, -22.0566) projected
  arc A89 (-158.2763, -22.0566) -> (-157.7496, -23.8531) centre (-80.0371, -0.0908) ccw projected
  line L89 (-157.7496, -23.8531) -> (-156.2317, -24.2885) projected
  arc A90 (-155.3656, -26.8631) -> (-156.2317, -24.2885) centre (-156.6867, -25.8745) ccw projected
  line L90 (-155.3656, -26.8631) -> (-156.3117, -28.1274) projected
  arc A91 (-156.3117, -28.1274) -> (-155.6456, -29.8771) centre (-80.0371, -0.0908) ccw projected
  line L91 (-155.6456, -29.8771) -> (-154.0983, -30.1921) projected
  arc A92 (-153.0329, -32.6908) -> (-154.0983, -30.1921) centre (-154.4274, -31.8089) ccw projected
  line L92 (-153.0329, -32.6908) -> (-153.8769, -34.0254) projected
  arc A93 (-153.8769, -34.0254) -> (-153.0755, -35.7174) centre (-80.0371, -0.0908) ccw projected
  line L93 (-153.0755, -35.7174) -> (-151.5082, -35.9101) projected
  arc A94 (-150.2501, -38.3175) -> (-151.5082, -35.9101) centre (-151.7095, -37.5477) ccw projected
  line L94 (-150.2501, -38.3175) -> (-150.9868, -39.7142) projected
  arc A95 (-150.9868, -39.7142) -> (-150.0552, -41.3381) centre (-80.0371, -0.0908) ccw projected
  line L95 (-150.0552, -41.3381) -> (-148.4776, -41.4072) projected
  arc A96 (-147.0344, -43.7085) -> (-148.4776, -41.4072) centre (-148.5498, -43.0556) ccw projected
  line L96 (-147.0344, -43.7085) -> (-147.6592, -45.1587) projected
  arc A97 (-147.6592, -45.1587) -> (-146.6031, -46.7045) centre (-80.0371, -0.0908) ccw projected
  line L97 (-146.6031, -46.7045) -> (-145.0249, -46.6496) projected
  arc A98 (-143.4057, -48.8306) -> (-145.0249, -46.6496) centre (-144.9676, -48.2986) ccw projected
  line L98 (-143.4057, -48.8306) -> (-143.9148, -50.3254) projected
  arc A99 (-143.9148, -50.3254) -> (-142.7406, -51.7835) centre (-80.0371, -0.0908) ccw projected
  line L99 (-142.7406, -51.7835) -> (-141.1716, -51.605) projected
  arc A100 (-139.3863, -53.6522) -> (-141.1716, -51.605) centre (-140.9851, -53.2444) ccw projected
  line L100 (-139.3863, -53.6522) -> (-139.7765, -55.1823) projected
  arc A101 (-139.7765, -55.1823) -> (-138.4915, -56.5438) centre (-80.0371, -0.0908) ccw projected
  line L101 (-138.4915, -56.5438) -> (-136.9414, -56.2427) projected
  arc A102 (-135.0009, -58.1435) -> (-136.9414, -56.2427) centre (-136.6268, -57.8625) ccw projected
  line L102 (-135.0009, -58.1435) -> (-135.2699, -59.6995) projected
  arc A103 (-135.2699, -59.6995) -> (-133.8821, -60.9561) centre (-80.0371, -0.0908) ccw projected
  line L103 (-133.8821, -60.9561) -> (-132.3604, -60.5343) projected
  arc A104 (-130.2767, -62.277) -> (-132.3604, -60.5343) centre (-131.9196, -62.1243) ccw projected
  line L104 (-130.2767, -62.277) -> (-130.4228, -63.8493) projected
  arc A105 (-130.4228, -63.8493) -> (-128.9407, -64.9931) centre (-80.0371, -0.0908) ccw projected
  line L105 (-128.9407, -64.9931) -> (-127.4567, -64.4532) projected
  arc A106 (-125.2428, -66.027) -> (-127.4567, -64.4532) centre (-126.8926, -66.0038) ccw projected
  line L106 (-125.2428, -66.027) -> (-125.265, -67.606) projected
  arc A107 (-125.265, -67.606) -> (-123.6977, -68.6299) centre (-80.0371, -0.0908) ccw projected
  line L107 (-123.6977, -68.6299) -> (-122.2607, -67.9753) projected
  arc A108 (-119.9301, -69.3706) -> (-122.2607, -67.9753) centre (-121.5767, -69.4768) ccw projected
  line L108 (-119.9301, -69.3706) -> (-119.8284, -70.9464) projected
  arc A109 (-119.8284, -70.9464) -> (-118.1856, -71.8442) centre (-80.0371, -0.0908) ccw projected
  line L109 (-118.1856, -71.8442) -> (-116.8044, -71.0788) projected
  arc A110 (-114.3715, -72.287) -> (-116.8044, -71.0788) centre (-116.0047, -72.5221) ccw projected
  line L110 (-114.3715, -72.287) -> (-114.1465, -73.8499) projected
  arc A111 (-114.1465, -73.8499) -> (-112.4383, -74.6161) centre (-80.0371, -0.0908) ccw projected
  line L111 (-112.4383, -74.6161) -> (-111.1214, -73.7447) projected
  arc A112 (-108.6012, -74.7583) -> (-111.1214, -73.7447) centre (-110.2109, -75.1208) ccw projected
  line L112 (-108.6012, -74.7583) -> (-108.2543, -76.2988) projected
  arc A113 (-108.2543, -76.2988) -> (-106.4912, -76.9286) centre (-80.0371, -0.0908) ccw projected
  line L113 (-106.4912, -76.9286) -> (-105.2468, -75.9565) projected
  arc A114 (-102.6548, -76.7692) -> (-105.2468, -75.9565) centre (-104.2311, -77.2569) ccw projected
  line L114 (-102.6548, -76.7692) -> (-102.1881, -78.2777) projected
  arc A115 (-102.1881, -78.2777) -> (-100.3811, -78.7673) centre (-80.0371, -0.0908) ccw projected
  line L115 (-100.3811, -78.7673) -> (-99.2167, -77.7006) projected
  arc A116 (-96.569, -78.3074) -> (-99.2167, -77.7006) centre (-98.1021, -78.9172) ccw projected
  line L116 (-96.569, -78.3074) -> (-95.9853, -79.7746) projected
  arc A117 (-95.9853, -79.7746) -> (-94.1455, -80.1209) centre (-80.0371, -0.0908) ccw projected
  line L117 (-94.1455, -80.1209) -> (-93.0684, -78.9662) projected
  arc A118 (-90.3812, -79.3633) -> (-93.0684, -78.9662) centre (-91.8618, -80.0916) ccw projected
  line L118 (-90.3812, -79.3633) -> (-89.6842, -80.7803) projected
  arc A119 (-89.6842, -80.7803) -> (-87.8229, -80.9811) centre (-80.0371, -0.0908) ccw projected
  line L119 (-87.8229, -80.9811) -> (-86.8397, -79.7454) projected
  arc A120 (-84.1297, -79.9306) -> (-86.8397, -79.7454) centre (-85.5485, -80.7727) ccw projected
  line L120 (-84.1297, -79.9306) -> (-83.3237, -81.2885) projected
  arc A121 (-83.3237, -81.2885) -> (-81.4523, -81.3426) centre (-80.0371, -0.0908) ccw projected
  line L121 (-81.4523, -81.3426) -> (-80.5691, -80.0336) projected
  arc A122 (-77.8529, -80.0055) -> (-80.5691, -80.0336) centre (-79.2013, -80.9564) ccw projected
  line L122 (-77.8529, -80.0055) -> (-76.9428, -81.296) projected
  arc A123 (-76.9428, -81.296) -> (-75.073, -81.2032) centre (-80.0371, -0.0908) ccw projected
  line L123 (-75.073, -81.2032) -> (-74.2952, -79.8289) projected
  arc A124 (-71.5896, -79.5878) -> (-74.2952, -79.8289) centre (-72.8593, -80.6416) ccw projected
  line L124 (-71.5896, -79.5878) -> (-70.5811, -80.8029) projected
  arc A125 (-70.5811, -80.8029) -> (-68.7243, -80.5636) centre (-80.0371, -0.0908) ccw projected
  line L125 (-68.7243, -80.5636) -> (-68.0568, -79.1326) projected
  arc A126 (-65.3784, -78.68) -> (-68.0568, -79.1326) centre (-66.5614, -79.8301) ccw projected
  line L126 (-65.3784, -78.68) -> (-64.2776, -79.8122) projected
  arc A127 (-64.2776, -79.8122) -> (-62.4453, -79.428) centre (-80.0371, -0.0908) ccw projected
  line L127 (-62.4453, -79.428) -> (-61.8921, -77.949) projected
  arc A128 (-59.2575, -77.2876) -> (-61.8921, -77.949) centre (-60.3467, -78.527) ccw projected
  line L128 (-59.2575, -77.2876) -> (-58.0714, -78.3299) projected
  arc A129 (-58.0714, -78.3299) -> (-56.2748, -77.8032) centre (-80.0371, -0.0908) ccw projected
  line L129 (-56.2748, -77.8032) -> (-55.8394, -76.2853) projected
  arc A130 (-53.2648, -75.4192) -> (-55.8394, -76.2853) centre (-54.2534, -76.7403) ccw projected
  line L130 (-53.2648, -75.4192) -> (-52.0005, -76.3653) projected
  arc A131 (-52.0005, -76.3653) -> (-50.2508, -75.6992) centre (-80.0371, -0.0908) ccw projected
  line L131 (-50.2508, -75.6992) -> (-49.9358, -74.1519) projected
  arc A132 (-47.4371, -73.0865) -> (-49.9358, -74.1519) centre (-48.319, -74.4811) ccw projected
  line L132 (-47.4371, -73.0865) -> (-46.1025, -73.9305) projected
  arc A133 (-46.1025, -73.9305) -> (-44.4105, -73.1292) centre (-80.0371, -0.0908) ccw projected
  line L133 (-44.4105, -73.1292) -> (-44.2178, -71.5619) projected
  arc A134 (-41.8104, -70.3037) -> (-44.2178, -71.5619) centre (-42.5802, -71.7632) ccw projected
  line L134 (-41.8104, -70.3037) -> (-40.4137, -71.0404) projected
  arc A135 (-40.4137, -71.0404) -> (-38.7898, -70.1088) centre (-80.0371, -0.0908) ccw projected
  line L135 (-38.7898, -70.1088) -> (-38.7207, -68.5312) projected
  arc A136 (-36.4194, -67.088) -> (-38.7207, -68.5312) centre (-37.0723, -68.6034) ccw projected
  line L136 (-36.4194, -67.088) -> (-34.9692, -67.7128) projected
  arc A137 (-34.9692, -67.7128) -> (-33.4234, -66.6567) centre (-80.0371, -0.0908) ccw projected
  line L137 (-33.4234, -66.6567) -> (-33.4783, -65.0786) projected
  arc A138 (-31.2973, -63.4593) -> (-33.4783, -65.0786) centre (-31.8293, -65.0212) ccw projected
  line L138 (-31.2973, -63.4593) -> (-29.8026, -63.9684) projected
  arc A139 (-29.8026, -63.9684) -> (-28.3444, -62.7942) centre (-80.0371, -0.0908) ccw projected
  line L139 (-28.3444, -62.7942) -> (-28.5229, -61.2253) projected
  arc A140 (-26.4757, -59.4399) -> (-28.5229, -61.2253) centre (-26.8835, -61.0387) ccw projected
  line L140 (-26.4757, -59.4399) -> (-24.9456, -59.8301) projected
  arc A141 (-24.9456, -59.8301) -> (-23.5841, -58.5452) centre (-80.0371, -0.0908) ccw projected
  line L141 (-23.5841, -58.5452) -> (-23.8852, -56.995) projected
  arc A142 (-21.9844, -55.0545) -> (-23.8852, -56.995) centre (-22.2655, -56.6804) ccw projected
  line L142 (-21.9844, -55.0545) -> (-20.4284, -55.3235) projected
  arc A143 (-20.4284, -55.3235) -> (-19.1718, -53.9357) centre (-80.0371, -0.0908) ccw projected
  line L143 (-19.1718, -53.9357) -> (-19.5936, -52.414) projected
  arc A144 (-17.8509, -50.3303) -> (-19.5936, -52.414) centre (-18.0036, -51.9733) ccw projected
  line L144 (-17.8509, -50.3303) -> (-16.2786, -50.4764) projected
  arc A145 (-16.2786, -50.4764) -> (-15.1348, -48.9943) centre (-80.0371, -0.0908) ccw projected
  line L145 (-15.1348, -48.9943) -> (-15.6747, -47.5104) projected
  arc A146 (-14.1009, -45.2964) -> (-15.6747, -47.5104) centre (-14.1242, -46.9462) ccw projected
  line L146 (-14.1009, -45.2964) -> (-12.5219, -45.3187) projected
  arc A147 (-12.5219, -45.3187) -> (-11.498, -43.7514) centre (-80.0371, -0.0908) ccw projected
  line L147 (-11.498, -43.7514) -> (-12.1526, -42.3144) projected
  arc A148 (-10.7573, -39.9837) -> (-12.1526, -42.3144) centre (-10.6511, -41.6303) ccw projected
  line L148 (-10.7573, -39.9837) -> (-9.1815, -39.8821) projected
  arc A149 (-9.1815, -39.8821) -> (-8.2837, -38.2392) centre (-80.0371, -0.0908) ccw projected
  line L149 (-8.2837, -38.2392) -> (-9.0491, -36.858) projected
  arc A150 (-7.8409, -34.4251) -> (-9.0491, -36.858) centre (-7.6058, -36.0583) ccw projected
  line L150 (-7.8409, -34.4251) -> (-6.278, -34.2001) projected
  arc A151 (-6.278, -34.2001) -> (-5.5118, -32.4919) centre (-80.0371, -0.0908) ccw projected
  line L151 (-5.5118, -32.4919) -> (-6.3832, -31.175) projected
  arc A152 (-5.3697, -28.6548) -> (-6.3832, -31.175) centre (-5.0071, -30.2645) ccw projected
  line L152 (-5.3697, -28.6548) -> (-3.8291, -28.3079) projected
  arc A153 (-3.8291, -28.3079) -> (-3.1993, -26.5449) centre (-80.0371, -0.0908) ccw projected
  line L153 (-3.1993, -26.5449) -> (-4.1714, -25.3004) projected
  arc A154 (-3.3587, -22.7084) -> (-4.1714, -25.3004) centre (-2.871, -24.2847) ccw projected
  line L154 (-3.3587, -22.7084) -> (-1.8502, -22.2417) projected
  arc A155 (-1.8502, -22.2417) -> (-1.3606, -20.4347) centre (-80.0371, -0.0908) ccw projected
  line L155 (-1.3606, -20.4347) -> (-2.4273, -19.2703) projected
  arc A156 (-1.8205, -16.6226) -> (-2.4273, -19.2703) centre (-1.2107, -18.1558) ccw projected
  line L156 (-1.8205, -16.6226) -> (-0.3533, -16.0389) projected
  arc A157 (-0.3533, -16.0389) -> (-0.007, -14.1991) centre (-80.0371, -0.0908) ccw projected
  line L157 (-0.007, -14.1991) -> (-1.1618, -13.122) projected
  arc A158 (-0.7646, -10.4348) -> (-1.1618, -13.122) centre (-0.0363, -11.9154) ccw projected
  line L158 (-0.7646, -10.4348) -> (0.6524, -9.7379) projected
  arc A159 (0.6524, -9.7379) -> (0.8532, -7.8765) centre (-80.0371, -0.0908) ccw projected
  line L159 (0.8532, -7.8765) -> (-0.3825, -6.8933) projected
  arc A160 (-1.0768, -4.9175) -> (-0.3825, -6.8933) centre (0.4734, -5.4827) ccw projected
  circle A161 centre (-80.0371, -0.0908) radius 5.5 projected
  circle A162 centre (-80.0371, -0.0908) radius 17.9
  line L160 (-80.0374, 17.8092) -> (-80.0374, 16.0092) construction
  line L161 (-80.0374, 17.8092) -> (-78.2374, 17.8092) construction
  arc A163 (-80.0374, 16.0092) -> (-78.2397, 17.7188) centre (-80.0374, 17.8092) ccw
  arc A164 (-81.8351, 17.7187) -> (-80.0374, 16.0092) centre (-80.0374, 17.8092) ccw
  arc A165 (-93.9803, 7.959) -> (-94.5619, 10.3707) centre (-95.5391, 8.859) ccw
  arc A166 (-96.3596, 7.2569) -> (-93.9803, 7.959) centre (-95.5391, 8.859) ccw
  arc A167 (-93.98, -8.141) -> (-96.3594, -7.4389) centre (-95.5389, -9.041) ccw
  arc A168 (-94.5616, -10.5526) -> (-93.98, -8.141) centre (-95.5389, -9.041) ccw
  arc A169 (-80.0369, -16.1908) -> (-81.8346, -17.9003) centre (-80.0369, -17.9908) ccw
  arc A170 (-78.2392, -17.9002) -> (-80.0369, -16.1908) centre (-80.0369, -17.9908) ccw
  arc A171 (-66.094, -8.1405) -> (-65.5124, -10.5522) centre (-64.5352, -9.0405) ccw
  arc A172 (-63.7147, -7.4384) -> (-66.094, -8.1405) centre (-64.5352, -9.0405) ccw
  arc A173 (-66.0943, 7.9595) -> (-63.7149, 7.2573) centre (-64.5354, 8.8595) ccw
  arc A174 (-65.5127, 10.3711) -> (-66.0943, 7.9595) centre (-64.5354, 8.8595) ccw
  dimension "d11" = 35.8
  dimension "d12" = 1.8
  dimension "d13" = 90
  dimension "d16" = 360
  constraints: 33 point on circle, 13 centre point, 8 coincident, 4 end point, 1 horizontal, 1 perpendicular, 1 vertical, 43 other
  measures "d11" diameter of A162
  measures "d12" distance of L160.start L160.end
  measures "d13" angle of L160 L161
ref_plane "作業平面4" through (35.15, 8.6756, -79.5656) normal (1, 0, 0) x (0, 0.1072674, -0.9942302)
sketch "スケッチ4" plane through (35.15, 8.6756, -79.5656) normal (1, 0, 0) x (0, 0.1072674, -0.9942302)
  arc A0 (-96.3596, 7.2569) -> (-93.9803, 7.959) centre (-95.5391, 8.859) ccw projected
  arc A1 (-93.9803, 7.959) -> (-94.5619, 10.3707) centre (-95.5391, 8.859) ccw projected
  circle A2 centre (-80.0371, -0.0908) radius 17.9 projected
  arc A3 (-81.8351, 17.7187) -> (-80.0374, 16.0092) centre (-80.0374, 17.8092) ccw projected
  arc A4 (-80.0374, 16.0092) -> (-78.2397, 17.7188) centre (-80.0374, 17.8092) ccw projected
  arc A5 (-65.5127, 10.3711) -> (-66.0943, 7.9595) centre (-64.5354, 8.8595) ccw projected
  arc A6 (-66.0943, 7.9595) -> (-63.7149, 7.2573) centre (-64.5354, 8.8595) ccw projected
  arc A7 (-66.094, -8.1405) -> (-65.5124, -10.5522) centre (-64.5352, -9.0405) ccw projected
  arc A8 (-63.7147, -7.4384) -> (-66.094, -8.1405) centre (-64.5352, -9.0405) ccw projected
  arc A9 (-80.0369, -16.1908) -> (-81.8346, -17.9003) centre (-80.0369, -17.9908) ccw projected
  arc A10 (-78.2392, -17.9002) -> (-80.0369, -16.1908) centre (-80.0369, -17.9908) ccw projected
  arc A11 (-94.5616, -10.5526) -> (-93.98, -8.141) centre (-95.5389, -9.041) ccw projected
  arc A12 (-93.98, -8.141) -> (-96.3594, -7.4389) centre (-95.5389, -9.041) ccw projected
  point P0 (-80.0371, -0.0908)
  constraints: 1 other
extrude "押し出し3" cut sketch "スケッチ4" along normal mid plane 82.905 contours A0 A1 A2 A3 A4 A5 A6 A8 A7 A10 A9 A11 A12